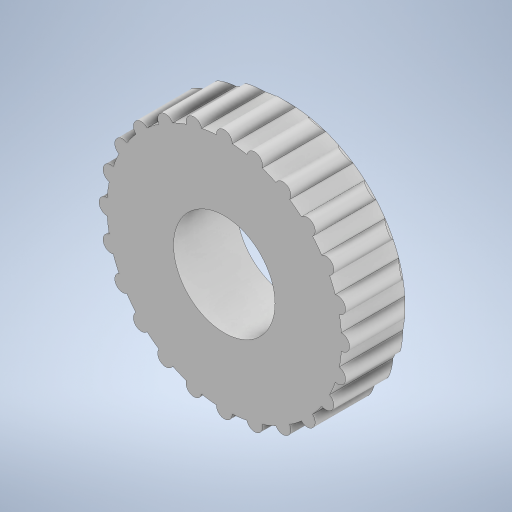
# Autodesk Inventor part: ATT_LED_BTM
Saved by Autodesk Inventor 2024 (Build 280153000, 153)
## iProperties
Created: 2024-11-27
Part Number: ATT_LED_BTM
Material: Типовые
Document SubType Name: Modeling
Designer: fm
Density: 1 g/cm^3
Appearance: По умолчанию
Author: fm
Autodesk Inventor part; units mm, degrees
ref_plane "YZ Plane" through (0, 0, 0) normal (1, 0, 0) x (0, 1, 0)
ref_plane "XZ Plane" through (0, 0, 0) normal (0, 1, 0) x (-1, 0, 0)
ref_plane "XY Plane" through (0, 0, 0) normal (0, 0, 1) x (1, 0, 0)
sketch "Эскиз1" plane through (0, 0, 0) normal (0, 0, 1) x (1, 0, 0)
  circle A0 centre (0, 0) radius 3.2
  circle A1 centre (0, 0) radius 7.4
  circle A2 centre (0, 0) radius 4
  line L0 (-2.54, 0) -> (2.54, 0) construction
  circle A3 centre (0, -7.4) radius 0.5
  circle A4 centre (1.915261, -7.147851) radius 0.5
  circle A5 centre (3.7, -6.408588) radius 0.5
  circle A6 centre (5.23259, -5.23259) radius 0.5
  circle A7 centre (6.408588, -3.7) radius 0.5
  circle A8 centre (7.147851, -1.915261) radius 0.5
  circle A9 centre (7.4, 0) radius 0.5
  circle A10 centre (7.147851, 1.915261) radius 0.5
  circle A11 centre (6.408588, 3.7) radius 0.5
  circle A12 centre (5.23259, 5.23259) radius 0.5
  circle A13 centre (3.7, 6.408588) radius 0.5
  circle A14 centre (1.915261, 7.147851) radius 0.5
  circle A15 centre (0, 7.4) radius 0.5
  circle A16 centre (-1.915261, 7.147851) radius 0.5
  circle A17 centre (-3.7, 6.408588) radius 0.5
  circle A18 centre (-5.23259, 5.23259) radius 0.5
  circle A19 centre (-6.408588, 3.7) radius 0.5
  circle A20 centre (-7.147851, 1.915261) radius 0.5
  circle A21 centre (-7.4, 0) radius 0.5
  circle A22 centre (-7.147851, -1.915261) radius 0.5
  circle A23 centre (-6.408588, -3.7) radius 0.5
  circle A24 centre (-5.23259, -5.23259) radius 0.5
  circle A25 centre (-3.7, -6.408588) radius 0.5
  circle A26 centre (-1.915261, -7.147851) radius 0.5
  point P0 (1.428202, 7.26087)
  point P1 (2.393576, 7.002199)
  point P2 (4.867294, 5.573997)
  point P3 (5.573997, 4.867294)
  point P4 (6.144102, 4.12432)
  point P5 (6.643816, 3.258789)
  point P6 (3.258789, 6.643816)
  point P7 (4.12432, 6.144102)
  point P8 (7.002199, 2.393576)
  point P9 (7.26087, 1.428202)
  point P10 (-0.499715, 7.383108)
  point P11 (0.499715, 7.383108)
  point P12 (-2.393576, 7.002199)
  point P13 (-1.428202, 7.26087)
  point P14 (-4.12432, 6.144102)
  point P15 (-3.258789, 6.643816)
  point P16 (-5.573997, 4.867294)
  point P17 (-4.867294, 5.573997)
  point P18 (-6.643816, 3.258789)
  point P19 (-6.144102, 4.12432)
  point P20 (-7.26087, 1.428202)
  point P21 (-7.002199, 2.393576)
  point P22 (-7.383108, -0.499715)
  point P23 (-7.383108, 0.499715)
  point P24 (-7.002199, -2.393576)
  point P25 (-7.26087, -1.428202)
  point P26 (-6.144102, -4.12432)
  point P27 (-6.643816, -3.258789)
  point P28 (-4.867294, -5.573997)
  point P29 (-5.573997, -4.867294)
  point P30 (-3.258789, -6.643816)
  point P31 (-4.12432, -6.144102)
  point P32 (-1.428202, -7.26087)
  point P33 (-2.393576, -7.002199)
  point P34 (-0.499715, -7.383108)
  point P35 (0.499715, -7.383108)
  point P36 (2.393576, -7.002199)
  point P37 (1.428202, -7.26087)
  point P38 (4.12432, -6.144102)
  point P39 (3.258789, -6.643816)
  point P40 (5.573997, -4.867294)
  point P41 (4.867294, -5.573997)
  point P42 (6.643816, -3.258789)
  point P43 (6.144102, -4.12432)
  point P44 (7.26087, -1.428202)
  point P45 (7.002199, -2.393576)
  point P46 (7.383108, 0.499715)
  point P47 (7.383108, -0.499715)
  dimension "d1" = 14.8
  dimension "d0" = 6.4
  dimension "d7" = 8
  dimension "d9" = 2.54
  dimension "d36" = 1
  dimension "d39" = 360
  constraints: 26 centre point, 2 coincident, 2 end point, 1 horizontal, 1 midpoint, 52 other
  measures "d0" diameter of A0
  measures "d7" diameter of A2
  measures "d9" distance of point (0, 0) L0.start
  measures "d36" diameter of A3
extrude "Выдавливание8" add sketch "Эскиз1" along normal blind 4 contours A1 A9 | A1 A9 | A9 A1 A8 A7 A6 A5 A4 A3 A26 A25 A24 A23 A22 A21 A20 A19 A18 A17 A16 A15 A14 A13 A12 A11 A10 | A10 A1 | A1 A10 | A8 A1 | A1 A8 | A11 A1 | A1 A11 | A7 A1 | A1 A7 | A12 A1 | A1 A12 | A6 A1 | A1 A6 | A13 A1 | A1 A13 | A5 A1 | A1 A5 | A14 A1 | A1 A14 | A4 A1 | A1 A4 | A15 A1 | A1 A15 | A3 A1 | A1 A3 | A16 A1 | A1 A16 | A26 A1 | A1 A26 | A17 A1 | A1 A17 | A25 A1 | A1 A25 | A18 A1 | A1 A18 | A24 A1 | A1 A24 | A19 A1 | A1 A19 | A23 A1 | A1 A23 | A20 A1 | A1 A20 | A22 A1 | A1 A22 | A21 A1 | A1 A21 | A2
sketch "Эскиз3" plane through (0, 0, 0) normal (1, 0, 0) x (0, 1, 0)
  line L0 (7.9, 0) -> (7.9, 4)
  line L1 (-7.9, 0) -> (-7.9, 4)
  line L2 (7.9, 0) -> (7.4, 0)
  line L3 (7.9, 0) -> (8.4, 0) construction
  line L4 (7.4, 0) -> (8.814214, 1.414214)
  line L5 (7.4, 0) -> (9.4, 0) construction
  line L6 (0, -0.8) -> (0, 4.8)
  point P0 (0, 0)
  point P1 (7.9, 0.5)
  dimension "d41" = 0.5
  dimension "d43" = 2
  dimension "d44" = 45
  constraints: 8 end point, 3 horizontal, 2 equal length
  measures "d41" distance of L0.start L2.end
  measures "d43" distance of L2.end L4.end
  measures "d44" angle of L5 L4
revolve "Вращение1" cut sketch "Эскиз3" angle 360 about axis through (0, 0, -10) along (0, 0, 1)
